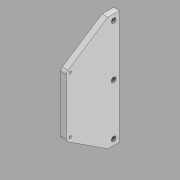
# Autodesk Inventor part: 202.001.05_Anbindung_Aktor
Saved by Autodesk Inventor 2021 (Build 250183000, 183)
## iProperties
Created: 2021-11-26
Part Number: 202.001.05_Anbindung_Aktor
Material: Generisch
Document SubType Name: Modeling
Designer: Oliver Ungerer
Density: 1 g/cm^3
Appearance: Vorgabe
Author: Oliver Ungerer
Autodesk Inventor part; units mm, degrees
ref_plane "YZ Plane" through (0, 0, 0) normal (1, 0, 0) x (0, 1, 0)
ref_plane "XZ Plane" through (0, 0, 0) normal (0, 1, 0) x (-1, 0, 0)
ref_plane "XY Plane" through (0, 0, 0) normal (0, 0, 1) x (1, 0, 0)
sketch "Skizze1" plane through (0, 0, 0) normal (1, 0, 0) x (0, 1, 0)
  line L0 (0, 0) -> (198, 0)
  line L1 (198, 0) -> (198, 92)
  line L2 (198, 92) -> (0, 92)
  line L3 (0, 92) -> (0, 0)
  dimension "d0" = 198
  dimension "d1" = 92
  constraints: 8 end point, 2 horizontal, 1 perpendicular, 1 vertical
  measures "d0" distance of L0.start L0.end
  measures "d1" distance of L0.end L1.end
extrude "Extrusion1" add sketch "Skizze1" along normal blind 10
sketch "Skizze2" plane through (10, 0, 0) normal (1, 0, 0) x (0, 0, -1)
  line L0 (-92, 0) -> (0, 0) projected
  line L1 (-85.5, 147.5) -> (-85.5, 50.5) construction
  line L2 (0, 0) -> (0, 198) projected
  dimension "d4" = 97
  dimension "d5" = 50.5
  dimension "d6" = 85.5
  constraints: 2 end point, 1 parallel
  measures "d4" distance of L1.end L1.start
  measures "d5" distance from line of L0 L1.end
  measures "d6" distance from line of L2 L1.start
hole "Bohrung1" at (10, 147.5, 85.5) at (10, 50.5, 85.5) direction (-1, 0, 0) diameter 4.2 depth 10 tip angle 118
sketch "Skizze3" plane through (10, 0, 0) normal (1, 0, 0) x (0, 0, -1)
  circle A0 centre (-85.5, 147.5) radius 2.1 projected
  circle A1 centre (-85.5, 50.5) radius 2.1 projected
  arc A2 (-92, 50.5) -> (-89.052, 45.0563) centre (-85.5, 50.5) ccw
  arc A3 (-89.052, 152.9437) -> (-92, 147.5) centre (-85.5, 147.5) ccw
  line L0 (0, 0) -> (0, 198) projected
  line L1 (0, 198) -> (-20, 198) construction
  line L2 (0, 0) -> (-20, 0) construction
  line L3 (-92, 0) -> (0, 0) projected
  line L4 (-20, 0) -> (-89.052, 45.0563)
  line L5 (-20, 198) -> (-89.052, 152.9437)
  line L6 (-92, 198) -> (-92, 0) projected
  line L7 (-20, 198) -> (-92, 198)
  line L8 (-92, 147.5) -> (-92, 198)
  line L9 (-92, 50.5) -> (-92, 0)
  line L10 (-92, 0) -> (-20, 0)
  dimension "d15" = 20
  constraints: 16 end point, 4 point on circle, 4 tangent, 3 point on line, 2 centre point, 2 coincident, 2 collinear, 1 horizontal, 1 perpendicular
  measures "d15" distance of L0.end L1.end
extrude "Extrusion2" cut sketch "Skizze3" against normal up to surface (10 mm away) contours A2 L4 L3 L6 | A3 L6 L7 L5
sketch "Skizze4" plane through (10, 0, 0) normal (1, 0, 0) x (0, 0, -1)
  line L0 (0, 0) -> (0, 198) projected
  line L1 (-20, 0) -> (0, 0) projected
  line L2 (0, 198) -> (-20, 198) projected
  line L3 (-92, 147.5) -> (-92, 50.5) projected
  line L4 (-92, 99) -> (0, 99)
  point P0 (-10, 10)
  point P1 (-10, 188)
  point P2 (-10, 99)
  dimension "d18" = 10
  dimension "d19" = 10
  dimension "d20" = 10
  constraints: 2 end point, 2 midpoint
  measures "d18" distance from line of point (-10, 10) L0
  measures "d19" distance from line of L1 point (-10, 10)
  measures "d20" distance from line of point (-10, 188) L2
hole "Bohrung2" at (10, 10, 10) at (10, 188, 10) at (10, 99, 10) direction (-1, 0, 0) diameter 4.5 end through all counterbore diameter 8 counterbore depth 5
